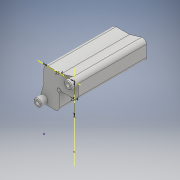
# Autodesk Inventor part: Jig2.1_1x1_Bolt_Pattern_PIN
Saved by Autodesk Inventor 2018 (Build 220112000, 112)
## iProperties
Created: 2018-12-01
Part Number: Jig2.1_1x1_Bolt_Pattern_PIN
Material: Generic
Document SubType Name: Modeling
Designer: Chris
Density: 1 g/cm^3
Appearance: Default
Author: Chris
Autodesk Inventor part; units mm, degrees
ref_plane "YZ Plane" through (0, 0, 0) normal (1, 0, 0) x (0, 1, 0)
ref_plane "XZ Plane" through (0, 0, 0) normal (0, 1, 0) x (-1, 0, 0)
ref_plane "XY Plane" through (0, 0, 0) normal (0, 0, 1) x (1, 0, 0)
sketch "Sketch1" plane through (0, 0, 0) normal (0, 1, 0) x (-1, 0, 0)
  line L0 (30.48, 0) -> (-5.08, 0) projected
  line L1 (0, -60.96) -> (0, 10.16) projected
  point P0 (0, 0)
  point P1 (0, 0)
  point P2 (0, -25.4)
  point P3 (0, -50.8)
  point P4 (25.4, 0)
  point P5 (25.4, -25.4)
  point P6 (25.4, -50.8)
  dimension "d2" = 25.4
  dimension "d5" = 25.4
  constraints: 1 coincident, 1 horizontal, 1 vertical, 5 other
  measures "d2" distance of point (0, 0) point (0, -25.4)
  measures "d5" distance of point (0, 0) point (25.4, 0)
sketch "Sketch2" plane through (0, 0, 0) normal (0, 1, 0) x (-1, 0, 0)
  arc A0 (0.9164, 3.0399) -> (-3.175, 0) centre (0, 0) ccw
  line L0 (0.9164, 3.0399) -> (11, 0)
  line L1 (11, 0) -> (25.4, 0)
  line L2 (12.7, -12.7) -> (-3.175, -12.7)
  line L3 (-3.175, -12.7) -> (-3.175, 0)
  line L4 (25.4, 0) -> (25.4, -14.4)
  line L5 (25.4, -14.4) -> (28.4399, -24.4836)
  arc A1 (25.4, -28.575) -> (28.4399, -24.4836) centre (25.4, -25.4) ccw
  line L6 (12.7, -12.7) -> (12.7, -28.575)
  line L7 (12.7, -28.575) -> (25.4, -28.575)
  point P0 (0, -50.8)
  point P1 (0, -25.4)
  dimension "d8" = 6.35
  dimension "d11" = 12.7
  dimension "d12" = 12.7
  dimension "d13" = 11
  dimension "d36" = 25.4
  dimension "d37" = 6.35
  dimension "d38" = 11
  dimension "d39" = 12.7
  dimension "d40" = 12.7
  constraints: 16 end point, 4 point on circle, 4 tangent, 2 centre point, 2 coincident, 1 horizontal, 1 perpendicular, 1 point on line, 1 vertical
  measures "d8" diameter of A0
  measures "d11" horizontal distance of point (0, 0) L2.start
  measures "d12" horizontal distance of point (0, 0) L2.start
  measures "d13" distance of point (0, 0) L0.end
  measures "d36" horizontal distance of point (0, 0) L4.end
  measures "d37" diameter of A1
  measures "d38" distance of A1.centre L4.end
  measures "d39" horizontal distance of point (0, 0) L2.start
  measures "d40" distance of L3.end L2.end
extrude "Extrusion1" add sketch "Sketch2" along normal blind 57.15
sketch "Sketch3" plane through (0, 0, 0) normal (0, -1, 0) x (1, 0, 0)
  circle A0 centre (0, 0) radius 3.175
  circle A1 centre (-25.4, -25.4) radius 3.175
  point P0 (-12.7, -12.7)
  dimension "d16" = 6.35
  dimension "d17" = 6.35
  constraints: 2 centre point, 2 coincident
  measures "d16" diameter of A0
  measures "d17" diameter of A1
extrude "Extrusion2" add sketch "Sketch3" along normal blind 5.588
sketch "Sketch4" plane through (0, 0, 0) normal (0, -1, 0) x (1, 0, 0)
  circle A0 centre (-12.7, -12.7) radius 1.5875
  point P0 (0, 0)
  dimension "d21" = 3.175
  constraints: 1 centre point, 1 coincident
  measures "d21" diameter of A0
extrude "Extrusion3" cut sketch "Sketch4" against normal through all
chamfer "Chamfer1" distance 0.5 angle 45 2 edges at (-3.175, -5.588, 0) (-28.575, -5.588, -25.4)
chamfer "Chamfer2" distance 0.5 angle 45 2 edges at (-11.1125, 28.575, -12.7) (-12.7, 28.575, -14.2875)
fillet "Fillet1" radius 3.175 2 edges at (3.175, 28.575, -12.7) (-25.4, 28.575, 0)
sketch "Sketch5" plane through (0, 57.15, 0) normal (0, 1, 0) x (1, 0, 0)
  line L0 (1.2744, 7.0637) -> (-10.8759, 7.0637) construction
  line L1 (-10.8759, 7.0637) -> (-10.8759, 12.3625) construction
  line L2 (-10.8759, 12.3625) -> (1.2744, 12.3625) construction
  line L3 (1.2744, 12.3625) -> (1.2744, 7.0637) construction
  line L4 (-23.4129, 5.226) -> (-12.7082, 5.226) construction
  line L5 (-12.7082, 5.226) -> (-12.7082, 1.3685) construction
  line L6 (-12.7082, 1.3685) -> (-23.4129, 1.3685) construction
  line L7 (-23.4129, 1.3685) -> (-23.4129, 5.226) construction
  point P0 (0, 0)
  constraints: 4 other
emboss "Emboss1" [suppressed]
fillet "Fillet2" radius 3.175 1 edges at (-12.7, 28.575, -28.575)
sketch "Sketch7" plane through (0, -5.588, 0) normal (0, -1, 0) x (1, 0, 0)
  circle A0 centre (0, 0) radius 2.675 projected
  circle A1 centre (-25.4, -25.4) radius 2.675 projected
  circle A2 centre (0, 0) radius 1.5875
  circle A3 centre (-25.4, -25.4) radius 3.175 projected
  circle A4 centre (-25.4, -25.4) radius 1.5875
  dimension "d42" = 3.175
  dimension "d43" = 3.175
  constraints: 2 centre point, 2 coincident
  measures "d42" diameter of A2
  measures "d43" diameter of A4
extrude "Extrusion4" cut sketch "Sketch7" against normal through all contours A2 | A4
body "Solid1"
